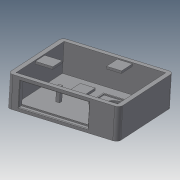
# Autodesk Inventor part: arduino case
Saved by Autodesk Inventor 2015 (Build 190159000, 159)
## iProperties
Created: 2017-05-03
Part Number: arduino case
Material: 일반
Document SubType Name: Modeling
Designer: gatew
Density: 1 g/cm^3
Appearance: 기본값
Author: gatew
Autodesk Inventor part; units mm, degrees
ref_plane "YZ Plane" through (0, 0, 0) normal (1, 0, 0) x (0, 1, 0)
ref_plane "XZ Plane" through (0, 0, 0) normal (0, 1, 0) x (-1, 0, 0)
ref_plane "XY Plane" through (0, 0, 0) normal (0, 0, 1) x (1, 0, 0)
sketch "스케치25" plane through (0, 0, 0) normal (0, 1, 0) x (-1, 0, 0)
  line L0 (35, 52.5) -> (-35, 52.5)
  line L1 (-35, 52.5) -> (-35, -52.5)
  line L2 (-35, -52.5) -> (35, -52.5)
  line L3 (35, -52.5) -> (35, 52.5)
  line L4 (35, 52.5) -> (-35, -52.5) construction
  line L5 (-35, 52.5) -> (35, -52.5) construction
  point P0 (0, 0)
  dimension "d167" = 70
  dimension "d168" = 105
  constraints: 12 end point, 2 midpoint, 2 parallel, 1 horizontal, 1 perpendicular
  measures "d167" distance of L2.end L1.end
  measures "d168" distance of L1.end L0.end
extrude "돌출20" add sketch "스케치25" along normal blind 28
fillet "모깎기9" radius 4 4 edges at (-35, 14, -52.5) (35, 14, -52.5) (35, 14, 52.5) (-35, 14, 52.5)
shell "쉘1" thickness 4 removed faces 1 at (11.6667, 28, 16.1667)
ref_plane "작업 평면6" through (-31, 17, 48.5) normal (0, 1, 0) x (1, 0, 0)
ref_plane "작업 평면7" through (-31, 19, 48.5) normal (0, 1, 0) x (1, 0, 0)
ref_plane "작업 평면8" through (-31, 20, 48.5) normal (0, 1, 0) x (1, 0, 0)
ref_plane "작업 평면9" through (0, 26, 0) normal (0, 1, 0) x (1, 0, 0)
sketch "스케치30" plane through (-31, 4, 48.5) normal (0, 1, 0) x (1, 0, 0)
  line L0 (0, 0) -> (0, 32) construction
  line L1 (0, 0) -> (0, 97) construction
  line L2 (0, 0) -> (51, 0) construction
  line L3 (0, 0) -> (62, 0) construction
  line L4 (51, 0) -> (51, 78) construction
  line L5 (51, 78) -> (27, 78) construction
  line L6 (27, 78) -> (27, 32) construction
  line L7 (27, 32) -> (0, 32) construction
  line L8 (6, 32) -> (9, 32)
  line L9 (9, 32) -> (9, 35)
  line L10 (9, 35) -> (6, 35)
  line L11 (6, 35) -> (6, 32)
  line L12 (6, 32) -> (9, 35) construction
  line L13 (9, 32) -> (6, 35) construction
  line L14 (51, 10) -> (54, 10)
  line L15 (54, 10) -> (54, 13)
  line L16 (54, 13) -> (51, 13)
  line L17 (51, 13) -> (51, 10)
  line L18 (51, 10) -> (54, 13) construction
  line L19 (54, 10) -> (51, 13) construction
  line L20 (31.5, 25) -> (51, 25)
  line L21 (51, 25) -> (51, 57.5)
  line L22 (51, 57.5) -> (31.5, 57.5)
  line L23 (31.5, 57.5) -> (31.5, 25)
  line L24 (31.5, 25) -> (51, 57.5) construction
  line L25 (51, 25) -> (31.5, 57.5) construction
  line L26 (32.5, 26) -> (50, 26)
  line L27 (50, 26) -> (50, 56.5)
  line L28 (50, 56.5) -> (32.5, 56.5)
  line L29 (32.5, 56.5) -> (32.5, 26)
  line L30 (62, 97) -> (62, 0) projected
  point P0 (31, 48.5)
  point P1 (0, 48.5)
  point P2 (7.5, 33.5)
  point P3 (52.5, 11.5)
  point P4 (41.25, 41.25)
  dimension "d207" = 32
  dimension "d210" = 24
  dimension "d211" = 3
  dimension "d212" = 3
  dimension "d213" = 6
  dimension "d214" = 0
  dimension "d216" = 3
  dimension "d217" = 3
  dimension "d218" = 0
  dimension "d219" = 10
  dimension "d225" = 0
  dimension "d227" = 19.5
  dimension "d228" = 1
  dimension "d229" = 32.5
  dimension "d289" = 25
  dimension "d290" = 8
  constraints: 56 end point, 8 parallel, 8 perpendicular, 6 midpoint, 3 horizontal, 2 point on line, 3 other
  measures "d207" distance of L0.start L0.end
  measures "d210" distance of L4.end L5.end
  measures "d211" distance of L10.end L9.end
  measures "d212" distance of L9.end L8.end
  measures "d213" distance between parallel lines of L1 L11
  measures "d214" distance between parallel lines of L7 L8
  measures "d216" distance of L16.end L15.end
  measures "d217" distance of L15.end L14.end
  measures "d218" distance between parallel lines of L4 L17
  measures "d219" distance between parallel lines of L3 L14
  measures "d225" distance between parallel lines of L4 L21
  measures "d227" distance of L20.start L20.end
  measures "d228" distance between parallel lines of L23 L29
  measures "d229" distance of L22.end L20.start
  measures "d289" distance between parallel lines of L2 L20
  measures "d290" distance between parallel lines of L30 L15
sketch "스케치31" plane through (-31, 4, 48.5) normal (0, 1, 0) x (1, 0, 0)
  point P0 (31, 48.5)
extrude "돌출25" add sketch "스케치30" along normal blind 12 contours L11 L10 L9 L8 | L17 L16 L15 L14
extrude "돌출26" add sketch "스케치30" along normal blind 1 contours L23 L22 L21 L20
sketch "스케치33" plane through (-31, 4, 48.5) normal (0, 1, 0) x (1, 0, 0)
  ellipse E0 centre (42, 40.5) end of major axis (48.5, 40.5) minor radius 9
  line L0 (32.5, 56.5) -> (50, 56.5) projected
  line L1 (50, 56.5) -> (50, 26) projected
  point P0 (31, 48.5)
  dimension "d232" = 6.5
  dimension "d233" = 9
  dimension "d234" = 16
  dimension "d235" = 8
  constraints: 2 other
  measures "d234" distance from line of L0 point (42, 40.5)
  measures "d235" distance from line of L1 point (42, 40.5)
extrude "돌출27" cut sketch "스케치33" against normal up to next
ref_plane "작업 평면10" through (0, 28.5, 0) normal (0, 1, 0) x (1, 0, 0)
sketch "스케치43" plane through (1.5, 4, 22.5) normal (0, 1, 0) x (1, 0, 0)
  point P0 (-1.5, 22.5)
sketch "스케치44" plane through (1.5, 4, 22.5) normal (0, 1, 0) x (1, 0, 0)
  ellipse E0 centre (9.5, 14.5) end of major axis (9.5, 23.5) minor radius 6.5 projected
  line L0 (0, 30.5) -> (0, 0) projected
  line L1 (0, 0) -> (17.5, 0) projected
  line L2 (17.5, 0) -> (17.5, 30.5) projected
  line L3 (17.5, 30.5) -> (0, 30.5) projected
  line L4 (17.5, 30.5) -> (17.5, 0)
  line L5 (0, 0) -> (17.5, 0)
  line L6 (17.5, 0) -> (17.5, 30.5)
  line L7 (17.5, 30.5) -> (0, 30.5)
  line L8 (0, 30.5) -> (0, 0)
  line L9 (17.5, 0) -> (17.5, 30.5)
  line L10 (0, 0) -> (0, 30.5)
  line L11 (0, 30.5) -> (17.5, 30.5) projected
  point P0 (-1.5, 22.5)
  constraints: 14 end point, 3 collinear, 3 perpendicular, 1 vertical, 1 other
sketch "스케치45" plane through (0, 0, 0) normal (0, -1, 0) x (1, 0, 0)
  line L0 (35, 75) -> (-35, 75)
  line L1 (-35, 75) -> (-35, -75)
  line L2 (-35, -75) -> (35, -75)
  line L3 (35, -75) -> (35, 75)
  line L4 (35, 75) -> (-35, -75) construction
  line L5 (-35, 75) -> (35, -75) construction
  point P0 (0, 0)
  dimension "d283" = 70
  dimension "d284" = 150
  constraints: 12 end point, 2 midpoint, 2 parallel, 1 horizontal, 1 perpendicular
  measures "d283" distance of L2.end L1.end
  measures "d284" distance of L1.end L0.end
extrude "돌출36" cut sketch "스케치45" against normal blind 2
sketch "스케치46" plane through (-31, 4, 48.5) normal (0, 1, 0) x (1, 0, 0)
  line L0 (50, 0) -> (0, 0)
  line L1 (50, 0) -> (50, 85)
  line L2 (50, 85) -> (26, 85)
  line L3 (0, 0) -> (0, 32)
  line L4 (0, 32) -> (26, 32)
  line L5 (26, 32) -> (26, 85)
  line L6 (0, 97) -> (0, 0) projected
  line L7 (62, 0) -> (0, 0) projected
  point P0 (25, 0)
  dimension "d291" = 50
  dimension "d292" = 85
  dimension "d293" = 24
  dimension "d294" = 32
  dimension "d295" = 0
  dimension "d296" = 0
  constraints: 12 end point, 3 perpendicular, 2 vertical, 1 horizontal
  measures "d291" distance of L0.start L0.end
  measures "d292" distance of L0.start L1.end
  measures "d293" distance of L1.end L2.end
  measures "d294" distance of L0.end L3.end
  measures "d295" distance between parallel lines of L6 L3
  measures "d296" distance between parallel lines of L7 L0
sketch "스케치47" plane through (-31, 4, 48.5) normal (0, 1, 0) x (1, 0, 0)
  point P0 (31, 48.5)
sketch "스케치48" plane through (-31, 4, 48.5) normal (0, 1, 0) x (1, 0, 0)
  line L0 (21, 74) -> (24, 74)
  line L1 (24, 74) -> (24, 77)
  line L2 (24, 77) -> (21, 77)
  line L3 (21, 77) -> (21, 74)
  line L4 (21, 74) -> (24, 77) construction
  line L5 (24, 74) -> (21, 77) construction
  line L6 (0, 97) -> (0, 0) projected
  line L7 (0, 97) -> (62, 97) projected
  point P0 (31, 48.5)
  point P1 (22.5, 75.5)
  point P2 (25, 97)
  dimension "d297" = 3
  dimension "d298" = 3
  dimension "d299" = 21
  dimension "d300" = 20
  constraints: 12 end point, 2 midpoint, 2 parallel, 1 horizontal, 1 perpendicular
  measures "d297" distance of L2.end L1.end
  measures "d298" distance of L1.end L0.end
  measures "d299" distance between parallel lines of L6 L3
  measures "d300" distance between parallel lines of L7 L2
extrude "돌출37" add sketch "스케치48" along normal blind 12
sketch "스케치50" plane through (-35, 28, -48.5) normal (-1, 0, 0) x (0, 0, 1)
  line L0 (5.8, -3) -> (60.8, -3)
  line L1 (60.8, -3) -> (60.8, -23)
  line L2 (60.8, -23) -> (5.8, -23)
  line L3 (5.8, -23) -> (5.8, -3)
  line L4 (5.8, -3) -> (60.8, -23) construction
  line L5 (60.8, -3) -> (5.8, -23) construction
  line L6 (97, 0) -> (0, 0) projected
  line L7 (0, -26) -> (0, 0) projected
  point P0 (48.5, -28)
  point P1 (33.3, -13)
  point P2 (42.5, 0)
  dimension "d312" = 55
  dimension "d313" = 20
  dimension "d315" = 3
  dimension "d316" = 5.8
  constraints: 12 end point, 2 midpoint, 2 parallel, 1 horizontal, 1 perpendicular
  measures "d312" distance of L1.end L2.end
  measures "d313" distance of L0.end L1.end
  measures "d315" distance between parallel lines of L6 L0
  measures "d316" distance between parallel lines of L7 L3
extrude "돌출39" cut sketch "스케치50" against normal up to next
sketch "스케치52" plane through (-35, 5, 12.3) normal (0, 0, -1) x (-1, 0, 0)
  line L0 (-2.9, 14.1) -> (-0.7, 14.1)
  line L1 (-0.7, 14.1) -> (-0.7, 7.9)
  line L2 (-0.7, 7.9) -> (-2.9, 7.9)
  line L3 (-2.9, 7.9) -> (-2.9, 14.1)
  line L4 (-2.9, 14.1) -> (-0.7, 7.9) construction
  line L5 (-0.7, 14.1) -> (-2.9, 7.9) construction
  line L6 (0, 23) -> (0, -3) projected
  line L7 (0, 0) -> (-4, 0) projected
  line L8 (-4, -1) -> (-66, -1) projected
  point P0 (-35, -5)
  point P1 (-1.8, 11)
  dimension "d319" = 2.2
  dimension "d320" = 6.2
  dimension "d321" = 0.7
  dimension "d353" = 12
  constraints: 12 end point, 2 midpoint, 2 parallel, 1 horizontal, 1 perpendicular
  measures "d319" distance of L1.end L2.end
  measures "d320" distance of L0.end L1.end
  measures "d321" distance between parallel lines of L6 L1
  measures "d353" distance from line of L8 point (-1.8, 11)
extrude "돌출40" cut sketch "스케치52" against normal blind 3
sketch "스케치53" plane through (-31, 4, 48.5) normal (1, 0, 0) x (0, 0, -1)
  line L0 (36.2, 21) -> (36.2, 20)
  line L1 (36.2, 21) -> (36.2, 1) projected
  line L2 (36.2, 20) -> (91.2, 20)
  line L3 (91.2, 1) -> (91.2, 21) projected
  line L4 (91.2, 20) -> (91.2, 21)
  line L5 (36.2, 21) -> (91.2, 21)
  line L6 (91.2, 21) -> (36.2, 21) projected
  line L7 (36.2, 1) -> (36.2, 2)
  line L8 (36.2, 2) -> (91.2, 2)
  line L9 (91.2, 2) -> (91.2, 1)
  line L10 (91.2, 1) -> (36.2, 1)
  line L11 (36.2, 1) -> (91.2, 1) projected
  point P0 (48.5, -4)
  dimension "d325" = 1
  dimension "d326" = 1
  constraints: 16 end point, 4 point on line, 2 collinear, 2 perpendicular, 2 vertical
  measures "d325" distance of L0.start L0.end
  measures "d326" distance of L1.end L7.end
extrude "돌출41" add sketch "스케치53" against normal blind 0.7 contours L5 L3 L2 L0 | L8 L3 L10 L1
ref_plane "작업 평면11" through (0, 27, 0) normal (0, 1, 0) x (1, 0, 0)
sketch "스케치54" plane through (0, 27, 0) normal (0, 1, 0) x (1, 0, 0)
  line L0 (-31, -52.5) -> (31, -52.5)
  line L1 (-31, -48.5) -> (31, -48.5)
  line L2 (-31, -6) -> (-17, -6)
  line L3 (-17, -6) -> (-17, 6)
  line L4 (-17, 6) -> (-31, 6)
  line L5 (-31, 6) -> (-31, -6)
  line L6 (-31, -6) -> (-17, 6) construction
  line L7 (-17, -6) -> (-31, 6) construction
  line L8 (-31, 48.5) -> (-31, -48.5)
  line L9 (-33.0051, 48.459) -> (-35, -48.5)
  line L10 (-6, 34.5) -> (-6, 48.5)
  line L11 (6, 34.5) -> (-6, 34.5)
  line L12 (6, 48.5) -> (6, 34.5)
  line L13 (-6, 48.5) -> (6, 48.5)
  line L14 (31, -6) -> (17, -6)
  line L15 (17, -6) -> (17, 6)
  line L16 (17, 6) -> (31, 6)
  line L17 (31, 6) -> (31, -6)
  line L18 (31, -6) -> (17, 6) construction
  line L19 (17, -6) -> (31, 6) construction
  point P0 (-24, 0)
  point P1 (24, 0)
  dimension "d333" = 12
  dimension "d334" = 10
  dimension "d335" = 0
  dimension "d336" = 14
  constraints: 40 end point, 4 midpoint, 2 parallel, 1 horizontal, 1 perpendicular
  measures "d333" distance of L3.end L2.end
  measures "d334" distance from line of L9 point (-24, 0)
  measures "d335" distance between parallel lines of L8 L5
  measures "d336" distance of L3.end L4.end
extrude "돌출42" add sketch "스케치54" against normal blind 2
chamfer "모따기7" distance 0.5 angle 45 6 edges at (-34.3, 16, 12.3) (-32.1, 16, 12.3) (-33.2, 19.1, 12.3) (-33.2, 12.9, 12.3) (-35, 15, -42.7) (-35, 15, 12.3)
chamfer "모따기8" distance 0.5 angle 45 2 edges at (-35, 25, -15.2) (-35, 5, -15.2)
sketch "스케치56" plane through (-31, 28, 52.5) normal (0, 0, 1) x (1, 0, 0)
  line L0 (-9.8317, 6.5279) -> (71.8317, 6.5279)
  line L1 (71.8317, 6.5279) -> (71.8317, -33.0144)
  line L2 (71.8317, -33.0144) -> (-9.8317, -33.0144)
  line L3 (-9.8317, -33.0144) -> (-9.8317, 6.5279)
  line L4 (-9.8317, 6.5279) -> (71.8317, -33.0144) construction
  line L5 (71.8317, 6.5279) -> (-9.8317, -33.0144) construction
  point P0 (31, -28)
  point P1 (31, -13.2433)
  constraints: 12 end point, 2 midpoint, 2 parallel, 1 horizontal, 1 perpendicular
extrude "돌출43" cut sketch "스케치56" against normal blind 20
sketch "스케치58" plane through (0, 28, 0) normal (0, 1, 0) x (1, 0, 0)
  line L0 (35, -32.5) -> (-35, -32.5)
  line L1 (-35, -32.5) -> (-35, -32.5)
  line L2 (-31, -36.5) -> (31, -36.5)
  line L3 (35, -32.5) -> (35, -32.5)
  arc A0 (31, -36.5) -> (35, -32.5) centre (31, -32.5) ccw
  arc A1 (-35, -32.5) -> (-31, -36.5) centre (-31, -32.5) ccw
  point P0 (0, 0)
  point P1 (-35, -36.5)
  dimension "d349" = 4
  dimension "d350" = 4
  constraints: 8 end point, 4 point on circle, 4 tangent, 3 perpendicular, 2 centre point, 2 point on line, 1 equal radius, 1 horizontal
  measures "d349" distance of L0.end point (-35, -36.5)
  measures "d350" radius of A0
extrude "돌출44" add sketch "스케치58" against normal up to surface (26 mm away)
